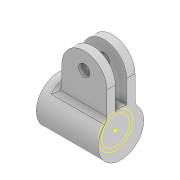
# Autodesk Inventor part: Hinge_2
Saved by Autodesk Inventor 2022 (Build 260153000, 153)
## iProperties
Created: 2022-07-08
Part Number: Hinge_2
Material: Generic
Document SubType Name: Modeling
Designer: dell
Density: 1 g/cm^3
Appearance: Default
Author: dell
Autodesk Inventor part; units mm, degrees
ref_plane "YZ Plane" through (0, 0, 0) normal (1, 0, 0) x (0, 1, 0)
ref_plane "XZ Plane" through (0, 0, 0) normal (0, 1, 0) x (-1, 0, 0)
ref_plane "XY Plane" through (0, 0, 0) normal (0, 0, 1) x (1, 0, 0)
sketch "Sketch1" plane through (0, 0, 0) normal (1, 0, 0) x (0, 1, 0)
  circle A0 centre (0, 0) radius 4.9
  circle A1 centre (0, 0) radius 6.1
  circle A2 centre (0, 0) radius 8.1
  dimension "d0" = 9.8
  dimension "d1" = 12.2
  dimension "d2" = 2
  constraints: 3 centre point, 2 coincident
  measures "d0" diameter of A0
  measures "d1" diameter of A1
  measures "d2" radial gap between concentric circles of A1 A2
extrude "Extrusion1" add sketch "Sketch1" along normal blind 20
sketch "Sketch2" plane through (20, 0, 0) normal (1, 0, 0) x (0, 0, -1)
  circle A0 centre (0, 0) radius 8.1 projected
  circle A1 centre (0, 0) radius 6.1 projected
extrude "Extrusion2" add sketch "Sketch2" along normal blind 2 contours A0 | A1
sketch "Sketch5" plane through (0, 0, 0) normal (0, 1, 0) x (-1, 0, 0)
  line L0 (-22, 8.1) -> (-22, -8.1) projected
  line L1 (-22, -5) -> (-6, -5)
  line L2 (-6, -5) -> (-6, -2)
  line L3 (-6, -2) -> (-22, -2)
  line L4 (-22, -2) -> (-22, -5)
  line L5 (-22, 5) -> (-6, 5)
  line L6 (-6, 5) -> (-6, 2)
  line L7 (-6, 2) -> (-22, 2)
  line L8 (-22, 2) -> (-22, 5)
  point P0 (0, 0)
  dimension "d23" = 16
  dimension "d24" = 2
  dimension "d25" = 2
  dimension "d26" = 3
  dimension "d27" = 3
  constraints: 16 end point, 4 parallel, 3 point on line, 2 horizontal, 2 perpendicular
  measures "d23" distance of L5.start L5.end
  measures "d24" distance from line of point (0, 0) L3
  measures "d25" distance from line of point (0, 0) L7
  measures "d26" distance between parallel lines of L7 L5
  measures "d27" distance between parallel lines of L3 L1
sketch "Sketch6" plane through (20, 0, 0) normal (-1, 0, 0) x (0, 0, 1)
  circle A0 centre (0, 0) radius 4.9 projected
  circle A1 centre (0, 0) radius 6.1 projected
extrude "Extrusion5" add sketch "Sketch5" along normal blind 24
sketch "Sketch7" plane through (22, 6.3726, -5) normal (0, 0, -1) x (-1, 0, 0)
  circle A0 centre (8, 11.6274) radius 2
  line L0 (0, 17.6274) -> (16, 17.6274) projected
  line L1 (16, 0) -> (16, 17.6274) projected
  arc A1 (16, 9.6274) -> (8, 17.6274) centre (8, 9.6274) ccw
  line L2 (0, 0) -> (0, 17.6274) projected
  arc A2 (8, 17.6274) -> (0, 9.6274) centre (8, 9.6274) ccw
  point P0 (22, -6.3726)
  dimension "d30" = 4
  dimension "d31" = 6
  dimension "d32" = 8
  constraints: 4 point on circle, 4 tangent, 3 centre point, 2 point on line, 1 midpoint
  measures "d30" diameter of A0
  measures "d31" distance from line of L0 A0.centre
  measures "d32" distance from line of L1 A0.centre
extrude "Extrusion6" cut sketch "Sketch7" against normal blind 100
fillet "Fillet2" radius 3 5 edges at (21, 6.3726, -5) (13, 6.3726, -5) (14, 6.3726, 5) (6, 7.2674, -3.577) (6, 7.2674, 3.577)
body "Solid1"
